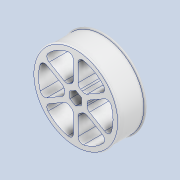
# Autodesk Inventor part: CUSTOM 4IN WHEEL
Saved by Autodesk Inventor 2021 (Build 250183000, 183)
## iProperties
Created: 2021-01-31
Part Number: CUSTOM 4IN WHEEL
Material: Aluminum 6061
Document SubType Name: Modeling
Designer: lucky
Mass: 226.262 g
Surface Area: 339.191 cm^2
Volume: 83.8007 cm^3
Density: 2.7 g/cm^3
Appearance: Aluminum - Flat
Author: lucky
Autodesk Inventor part; units mm, degrees
ref_plane "YZ Plane" through (0, 0, 0) normal (1, 0, 0) x (0, 1, 0)
ref_plane "XZ Plane" through (0, 0, 0) normal (0, 1, 0) x (-1, 0, 0)
ref_plane "XY Plane" through (0, 0, 0) normal (0, 0, 1) x (1, 0, 0)
sketch "Sketch1" plane through (0, 0, 0) normal (1, 0, 0) x (0, 1, 0)
  line L0 (0, 15.5575) -> (45.72, 15.5575)
  line L1 (45.72, 15.5575) -> (45.72, -15.5575)
  line L2 (45.72, -15.5575) -> (0, -15.5575)
  line L3 (0, -15.5575) -> (0, 15.5575)
  arc A0 (45.72, 13.0175) -> (45.72, 15.5575) centre (45.72, 14.2875) ccw
  arc A1 (45.72, -15.5575) -> (45.72, -13.0175) centre (45.72, -14.2875) ccw
  line L4 (45.72, 13.0175) -> (50.8, 13.0175)
  line L5 (50.8, 13.0175) -> (50.8, -13.0175)
  line L6 (50.8, -13.0175) -> (45.72, -13.0175)
  line L7 (45.72, -13.0175) -> (45.72, 13.0175)
  point P0 (0, 0)
  point P1 (45.72, 0)
  point P2 (0, 0)
  dimension "d0" = 1.27
  dimension "d1" = 1.27
  dimension "d2" = 45.72
  dimension "d3" = 26.035
  dimension "d4" = 5.08
  constraints: 16 end point, 4 parallel, 4 point on circle, 3 tangent, 2 centre point, 2 horizontal, 2 midpoint, 2 perpendicular, 2 point on line, 1 coincident, 1 horizontal alignment
  measures "d0" radius of A1
  measures "d1" radius of A0
  measures "d2" distance between parallel lines of L3 L1
  measures "d3" distance of A1.end L4.start
  measures "d4" distance between parallel lines of L1 L5
revolve "Revolution1" add sketch "Sketch1" angle 360 about axis through (0, 0, -15.5575) along (0, 0, 1) contours L0 L1 L2 L3 | A0 L1 | L1 A1
sketch "Sketch2" plane through (0, 0, 15.5575) normal (0, 0, 1) x (1, 0, 0)
  line L0 (-6.35, 3.6662) -> (0, 7.3323)
  line L1 (0, 7.3323) -> (6.35, 3.6662)
  line L2 (6.35, 3.6662) -> (6.35, -3.6662)
  line L3 (6.35, -3.6662) -> (0, -7.3323)
  line L4 (0, -7.3323) -> (-6.35, -3.6662)
  line L5 (-6.35, -3.6662) -> (-6.35, 3.6662)
  point P0 (0, 0)
  point P1 (0, 0)
  point P2 (6.35, 0)
  dimension "d6" = 12.7
  constraints: 12 end point, 1 coincident, 1 horizontal alignment, 1 midpoint, 13 other
  measures "d6" distance between parallel lines of L0 L3
extrude "Extrusion1" cut sketch "Sketch2" against normal through all
sketch "Sketch3" plane through (0, 0, 15.5575) normal (0, 0, 1) x (1, 0, 0)
  circle A0 centre (0, 0) radius 12.5
  circle A1 centre (0, 0) radius 45.72 construction
  circle A2 centre (0, 0) radius 40.72
  line L0 (0, -12.5) -> (0, -40.72)
  line L1 (6.35, -3.6662) -> (0, -7.3323) projected
  line L2 (0, -7.3323) -> (-6.35, -3.6662) projected
  line L3 (-6.35, -3.6662) -> (-6.35, 3.6662) projected
  line L4 (-6.35, 3.6662) -> (0, 7.3323) projected
  line L5 (0, 7.3323) -> (6.35, 3.6662) projected
  line L6 (6.35, 3.6662) -> (6.35, -3.6662) projected
  circle A3 centre (0, 0) radius 45.72 projected
  line L7 (0, 0) -> (35.2646, -20.36)
  line L8 (0, 0) -> (35.2646, 20.36)
  line L9 (0, 0) -> (0, 40.72)
  line L10 (0, 0) -> (-35.2646, 20.36)
  line L11 (0, 0) -> (-35.2646, -20.36)
  line L12 (-11.8566, 3.9587) -> (-36.448, 18.1565)
  line L13 (-9.3566, 8.2888) -> (-33.948, 22.4867)
  line L14 (-11.8566, -3.9587) -> (-36.448, -18.1565)
  line L15 (-9.3566, -8.2888) -> (-33.948, -22.4867)
  line L16 (-2.5, -12.2474) -> (-2.5, -40.6432)
  line L17 (2.5, -12.2474) -> (2.5, -40.6432)
  line L18 (9.3566, -8.2888) -> (33.948, -22.4867)
  line L19 (11.8566, -3.9587) -> (36.448, -18.1565)
  line L20 (11.8566, 3.9587) -> (36.448, 18.1565)
  line L21 (9.3566, 8.2888) -> (33.948, 22.4867)
  line L22 (2.5, 12.2474) -> (2.5, 40.6432)
  line L23 (-2.5, 12.2474) -> (-2.5, 40.6432)
  point P0 (-36.448, -18.1565)
  dimension "d9" = 25
  dimension "d10" = 5
  dimension "d13" = 2.5
  dimension "d14" = 5
  dimension "d17" = 360
  constraints: 36 end point, 5 point on line, 3 point on circle, 2 parallel, 2 vertical, 1 centre point, 1 coincident, 47 other
  measures "d9" diameter of A0
  measures "d13" distance between parallel lines of L13 L10
  measures "d14" distance between parallel lines of L13 L12
extrude "Extrusion2" cut sketch "Sketch3" against normal through all contours A0 L20 A2 L19 | A0 L22 A2 L21 | L18 A2 L17 A0 | A0 L13 A2 L23 | L16 A2 L15 A0 | A0 L14 A2 L12
fillet "Fillet1" radius 5 2 edges at (-33.948, 22.4867, 0) (-36.448, 18.1565, 0)
pattern_circular "Circular Pattern1" count 6 over 360 about axis through (0, 0, -10) along (0, 0, 1) of "Fillet1"
fillet "Fillet2" radius 5 2 edges at (9.3566, 8.2888, 0) (11.8566, 3.9587, 0)
pattern_circular "Circular Pattern2" count 6 over 360 about axis through (0, 0, -10) along (0, 0, 1) of "Fillet2"
equation "\"d1\" = d0"
body "Solid1"
